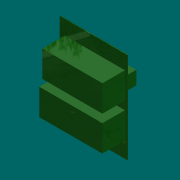
# Autodesk Inventor part: pcb
Saved by Autodesk Inventor 2020 (Build 240168000, 168)
## iProperties
Created: 2025-01-02
Part Number: pcb
Material: Plastica ABS
Document SubType Name: Modeling
Designer: Nicola Milia
Density: 1.06 g/cm^3
Appearance: Liscia - Bianco
Author: Nicola Milia
Autodesk Inventor part; units mm, degrees
ref_plane "YZ Plane" through (0, 0, 0) normal (1, 0, 0) x (0, 1, 0)
ref_plane "XZ Plane" through (0, 0, 0) normal (0, 1, 0) x (-1, 0, 0)
ref_plane "XY Plane" through (0, 0, 0) normal (0, 0, 1) x (1, 0, 0)
sketch "Schizzo1" plane through (0, 0, 0) normal (0, 0, 1) x (1, 0, 0)
  line L0 (0, 0) -> (90, 0)
  line L1 (90, 0) -> (90, -121)
  line L2 (90, -121) -> (0, -121)
  line L3 (0, -121) -> (0, 0)
  dimension "d0" = 90
  dimension "d1" = 121
  constraints: 8 end point, 2 parallel, 1 horizontal, 1 perpendicular
  measures "d0" distance of L1.end L2.end
  measures "d1" distance of L0.end L1.end
extrude "Estrusione1" add sketch "Schizzo1" along normal blind 1
sketch "Schizzo2" plane through (0, 0, 0) normal (0, 0, -1) x (-1, 0, 0)
  line L0 (-90, 0) -> (-90, -32)
  line L1 (-90, -121) -> (-90, 0) projected
  line L2 (-81, -32) -> (-66, -32)
  line L3 (-66, -32) -> (-66, -50)
  line L4 (-66, -50) -> (-81, -50)
  line L5 (-81, -50) -> (-81, -32)
  line L6 (-90, 0) -> (-90, -40)
  line L7 (-51, -40) -> (-29, -40)
  line L8 (-29, -40) -> (-29, -70)
  line L9 (-29, -70) -> (-51, -70)
  line L10 (-51, -70) -> (-51, -40)
  dimension "d10" = 22
  dimension "d11" = 30
  constraints: 20 end point, 4 parallel, 2 horizontal, 2 perpendicular, 2 point on line
  measures "d10" distance of L8.end L9.end
  measures "d11" distance of L7.end L8.end
extrude "Estrusione2" add sketch "Schizzo2" along normal blind 20
sketch "Schizzo3" plane through (0, 0, 1) normal (0, 0, 1) x (1, 0, 0)
  line L0 (90, -121) -> (90, 0) projected
  line L1 (90, 0) -> (90, -19)
  line L2 (87, -19) -> (7, -19)
  line L3 (7, -19) -> (7, -54)
  line L4 (7, -54) -> (87, -54)
  line L5 (87, -54) -> (87, -19)
  line L6 (90, -121) -> (90, -100)
  line L7 (87, -100) -> (3, -100)
  line L8 (3, -100) -> (3, -65)
  line L9 (3, -65) -> (87, -65)
  line L10 (87, -65) -> (87, -100)
  dimension "d16" = 80
  dimension "d17" = 35
  dimension "d19" = 84
  dimension "d20" = 35
  constraints: 20 end point, 4 parallel, 2 horizontal, 2 perpendicular, 2 point on line
  measures "d16" distance of L4.end L3.end
  measures "d17" distance of L3.end L2.end
  measures "d19" distance of L8.end L9.end
  measures "d20" distance of L7.end L8.end
extrude "Estrusione3" add sketch "Schizzo3" along normal blind 30
sketch "Schizzo4" plane through (0, 0, 1) normal (0, 0, 1) x (1, 0, 0)
  line L0 (90, -121) -> (90, 0) projected
  line L1 (90, 0) -> (90, -6)
  circle A0 centre (86, -6) radius 2
  circle A1 centre (4, -6) radius 2
  circle A2 centre (86, -106) radius 2
  circle A3 centre (4, -106) radius 2
  dimension "d28" = 4
  dimension "d32" = 4
  dimension "d33" = 4
  constraints: 4 centre point, 3 coincident, 2 end point, 1 point on line
  measures "d28" diameter of A1
  measures "d32" diameter of A2
  measures "d33" diameter of A3
extrude "Estrusione4" cut sketch "Schizzo4" against normal up to surface (1 mm away)
